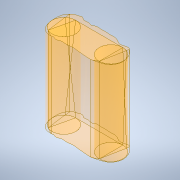
# Autodesk Inventor part: Kapton
Saved by Autodesk Inventor 2022 (Build 260153070, 153G)
## iProperties
Created: 2021-07-29
Part Number: Kapton
Material: Generic
Document SubType Name: Modeling
Designer: LJ
Density: 1 g/cm^3
Appearance: Default
Author: LJ
Autodesk Inventor part; units mm, degrees
ref_plane "Work Plane1" through (-0.6489, 57.7553, -49.1793) normal (0.0017309, 0.9999946, 0.0027762) x (0.9999985, -0.0017309, -0.0000024)
sketch "Sketch1" plane through (-0.6489, 57.7553, -49.1793) normal (0.0017309, 0.9999946, 0.0027762) x (0.9999985, -0.0017309, -0.0000024)
  circle A0 centre (0, 0) radius 9 projected
  line L0 (19.0189, 12.175) -> (12.9094, 12.175) projected
  line L1 (26.1347, 12.175) -> (20.0252, 12.175) projected
  circle A1 centre (36, 0) radius 9 projected
  circle A2 centre (18, 0) radius 9 projected
  spline S0 degree 4 poles (0, 0) (-0.6553, 0.9393) (-1.8109, 1.7925) (-2.0777, 3.7738) (-1.6084, 5.5868) (0.0105, 8.7964) (0.9505, 10.5382) (0.6689, 11.8602) (-0.5773, 12.0562) (-2.1364, 11.7342) (-4.3227, 10.9668) (-10.5073, 7.8875) (9.1877, 12.4202) (9.2116, 9.9398) knots 0 0 0 0 0 0.167802 0.242622 0.320476 0.395216 0.465981 0.526639 0.586559 0.652501 0.714955 1 1 1 1 1
  spline S1 degree 3 poles (35.4103, 0.0004) (35.5053, 0.524) (35.6027, 1.0612) (35.7334, 1.701) (35.99, 2.9576) (36.3593, 4.5369) (36.6244, 5.9708) (36.7554, 6.679) (36.8608, 7.3512) (36.9147, 7.9277) (36.9673, 8.4903) (36.9707, 8.9611) (36.9028, 9.2875) (36.8521, 9.5311) (36.762, 9.6946) (36.6361, 9.8005) (36.389, 10.0085) (36.0016, 9.9887) (35.5014, 9.8829) (34.889, 9.7534) (34.1057, 9.4918) (33.2228, 9.3567) (32.3613, 9.2249) (31.4183, 9.2115) (30.4339, 9.5143) (29.8991, 9.6789) (29.2864, 9.9624) (28.6807, 10.2059) (28.3816, 10.3262) (28.0815, 10.437) (27.7825, 10.5121) (27.4908, 10.5853) (27.1939, 10.6199) (26.945, 10.5735) (26.7256, 10.5326) (26.5741, 10.4399) (26.4467, 10.3351) (26.3224, 10.2328) (26.2215, 10.1171) (26.1249, 10.0075) knots 0 0 0 0 0.19652 0.19652 0.19652 0.582438 0.582438 0.582438 0.773039 0.773039 0.773039 0.959041 0.959041 0.959041 1.097848 1.097848 1.097848 1.370415 1.370415 1.370415 1.704123 1.704123 1.704123 2.029777 2.029777 2.029777 2.206716 2.206716 2.206716 2.294104 2.294104 2.294104 2.379384 2.379384 2.379384 2.454566 2.454566 2.454566 2.527933 2.527933 2.527933 2.527933 projected
  spline S2 degree 4 poles (18, 0) (19.219, -4.6198) (19.0867, -7.2448) (20.0738, -9.5935) (21.8548, -9.2534) (22.8608, -8.7189) (24.3983, -7.9162) (26.6917, -7.7224) (27.5292, -6.6832) (28.0308, -6.9813) (29.1474, -9.3707) (30.1409, -10.5959) (30.8392, -10.3204) (31.406, -9.5273) (32.8657, -2.3393) (33.0213, -3.9488) (34.3133, -0.7406) (36, 0) knots 0 0 0 0 0 0.198178 0.245011 0.293097 0.34823 0.403604 0.454446 0.508041 0.557208 0.603331 0.65184 0.7072 0.763584 0.826147 1 1 1 1 1
  spline S3 degree 4 poles (0, 0) (0.316, -1.3141) (-0.4427, -2.1492) (1.5587, -4.8996) (1.1525, -5.5021) (6.9051, -10.347) (5.2306, -9.9563) (5.4718, -9.4308) (4.7958, -8.7149) (4.8713, -8.5892) (6.0233, -7.3868) (6.4249, -6.4273) (7.496, -5.0511) (7.9624, -4.7173) (8.5564, -4.544) (9.1281, -4.9199) (9.5442, -5.4892) (10.5497, -8.0062) (11.3864, -8.8266) (11.913, -9.0938) (12.5739, -9.1265) (13.2529, -8.8682) (14.0483, -8.3031) (14.9715, -7.3561) (15.9318, -6.1181) (17.1481, -4.1239) (17.8173, -2.3655) (17.8952, -1.0974) (18, 0) knots 0 0 0 0 0 0.106192 0.157046 0.202296 0.242489 0.278377 0.299002 0.324044 0.354605 0.389092 0.425776 0.458865 0.486598 0.510804 0.543347 0.579427 0.615676 0.650761 0.678071 0.704423 0.734584 0.769524 0.808892 0.851075 0.893896 1 1 1 1 1
  line L2 (45, 0) -> (-9, 0) construction
  line L3 (36.017, -8.983) -> (-0.017, -8.983)
  line L4 (-0.017, 8.983) -> (36.017, 8.983)
  arc A3 (36.017, -8.983) -> (36.017, 8.983) centre (36.017, 0) ccw
  arc A4 (-0.017, 8.983) -> (-0.017, -8.983) centre (-0.017, 0) ccw
  spline S4 degree 4 poles (36.017, -8.983) (30.9958, -11.8975) (32.9255, -10.9101) (20.3119, -10.7814) (17.0217, -9.4088) (11.9966, -11.0587) (7.7415, -9.3427) (4.9899, -13.2783) (-0.7034, -7.4236) (4.6474, -13.4212) (-4.0003, -8.0516) knots 0 0 0 0 0 0.248405 0.34954 0.4777 0.586934 0.689222 0.769465 1 1 1 1 1
  line L5 (33.2745, -11.2682) -> (27.229, -10.9748) construction
  arc A5 (27.87, -10.8242) -> (32.6511, -11.0562) centre (31.021, 4.731) ccw construction
  spline S5 degree 4 poles (39.4127, 8.3165) (40.3947, 14.1433) (33.3903, 7.9791) (31.0784, 10.9351) (26.568, 13.0803) (22.0016, 12.3238) (19.3951, 13.1286) (15.2242, 12.4193) (10.9289, 13.6735) (10.0964, 10.5112) (5.6837, 13.436) (3.1602, 10.8421) (0.6242, 14.7157) (-1.5277, 12.7493) (-4.2485, 12.8468) (-8.0804, 10.3045) (-5.1576, 8.6318) (-5.9436, 6.7582) knots 0 0 0 0 0 0.164251 0.230539 0.292753 0.357884 0.423213 0.483129 0.544452 0.602591 0.659384 0.716439 0.769779 0.822475 0.871652 1 1 1 1 1
  point P0 (0.7487, -49.3395)
  point P1 (-1.1248, 1.4068)
  point P2 (-1.7551, 2.6503)
  point P3 (-1.8869, 3.9631)
  point P4 (-1.5342, 5.4984)
  point P5 (0.1303, 9.0153)
  point P6 (0.7446, 10.8943)
  point P7 (0.4337, 11.6763)
  point P8 (-0.4454, 11.9522)
  point P9 (-1.9244, 11.748)
  point P10 (-3.6466, 11.1412)
  point P11 (-5.2484, 10.192)
  point P12 (-4.8281, 9.9378)
  point P13 (19.4937, -7.2805)
  point P14 (20.2025, -8.8191)
  point P15 (20.9141, -9.2849)
  point P16 (21.7005, -9.2325)
  point P17 (22.6829, -8.8114)
  point P18 (24.5254, -8.0465)
  point P19 (26.8142, -7.3575)
  point P20 (27.5256, -6.9369)
  point P21 (27.9025, -7.0716)
  point P22 (29.3016, -9.4309)
  point P23 (30.2518, -10.3642)
  point P24 (30.6575, -10.3112)
  point P25 (31.1154, -9.766)
  point P26 (32.4478, -4.8226)
  point P27 (33.0116, -3.3798)
  point P28 (33.7624, -2.1885)
  point P29 (0.1165, -1.7118)
  point P30 (0.4378, -3.1699)
  point P31 (1.1027, -4.6194)
  point P32 (2.0695, -6.0716)
  point P33 (5.441, -9.7641)
  point P34 (5.6866, -9.9388)
  point P35 (5.2926, -9.3609)
  point P36 (4.9377, -8.8207)
  point P37 (4.9168, -8.6025)
  point P38 (5.6622, -7.7066)
  point P39 (6.6193, -6.2565)
  point P40 (7.6429, -4.9923)
  point P41 (8.0944, -4.7038)
  point P42 (8.5096, -4.6419)
  point P43 (8.9285, -4.8206)
  point P44 (9.398, -5.3741)
  point P45 (10.7591, -8.0516)
  point P46 (11.559, -8.8787)
  point P47 (12.0061, -9.0622)
  point P48 (12.5129, -9.0802)
  point P49 (13.1221, -8.8868)
  point P50 (13.8878, -8.382)
  point P51 (14.8388, -7.4545)
  point P52 (15.86, -6.1538)
  point P53 (16.7814, -4.6401)
  point P54 (17.4543, -3.102)
  point P55 (17.8169, -1.6352)
  point P56 (18, 0)
  point P57 (30.2518, -11.1215)
  point P58 (20.8791, -10.3343)
  point P59 (16.3717, -9.9691)
  point P60 (11.5107, -10.3427)
  point P61 (7.5994, -10.3924)
  point P62 (4.8814, -11.175)
  point P63 (2.404, -10.3272)
  point P64 (2.0502, -10.3236)
  point P65 (37.3714, 11.1319)
  point P66 (32.4445, 10.1835)
  point P67 (29.6646, 11.3962)
  point P68 (26.4295, 12.6021)
  point P69 (22.2745, 12.6345)
  point P70 (19.1979, 12.8254)
  point P71 (14.8368, 12.8262)
  point P72 (11.3002, 12.6682)
  point P73 (9.5875, 11.7437)
  point P74 (5.94, 12.3522)
  point P75 (3.0221, 12.1719)
  point P76 (0.4369, 13.622)
  point P77 (-1.5349, 13.1224)
  point P78 (-3.6471, 12.5265)
  point P79 (-5.9261, 11.1402)
  point P80 (-6.2045, 9.4639)
  point P81 (39.4145, 8.3271)
  point P82 (0.5527, 8.983)
  point P83 (17.4473, 8.983)
  point P84 (18.5527, 8.983)
  point P85 (35.4473, 8.983)
  point P86 (-3.9193, -8.1018)
  point P87 (35.9877, -9)
  constraints: 12 point on circle, 10 end point, 4 tangent, 3 centre point, 3 midpoint, 2 point on line, 1 horizontal, 1 parallel, 152 other
sketch "Sketch2" plane through (0, 0, 0) normal (1, 0, 0) x (0, 1, 0)
  point P0 (0, 0)
ref_plane "Work Plane2" through (35.2391, -7.0067, -49.359) normal (-0.0017309, -0.9999946, -0.0027762) x (-0.9999985, 0.0017309, 0.0000024)
sketch "Sketch3" plane through (35.2391, -7.0067, -49.359) normal (-0.0017309, -0.9999946, -0.0027762) x (-0.9999985, 0.0017309, 0.0000024)
  circle A0 centre (0, 0) radius 9
  line L0 (36.017, 8.983) -> (-0.017, 8.983) projected
  circle A1 centre (36, 0) radius 9
  line L1 (-0.017, -8.983) -> (36.017, -8.983) projected
  spline S0 degree 4 poles (-0.017, -8.983) (5.0042, -11.8975) (3.0745, -10.9101) (15.6881, -10.7814) (18.9783, -9.4088) (24.0034, -11.0587) (28.2585, -9.3427) (31.0101, -13.2783) (36.7034, -7.4236) (31.3526, -13.4212) (40.0003, -8.0516) knots 0 0 0 0 0 0.248405 0.34954 0.4777 0.586934 0.689222 0.769465 1 1 1 1 1 projected
  point P0 (35.2513, -49.3395)
  constraints: 2 centre point
sketch3d "3D Sketch1"
sketch "Sketch4" plane through (-0.6489, 57.7553, -49.1793) normal (0.0017309, 0.9999946, 0.0027762) x (0.9999985, -0.0017309, -0.0000024)
  spline S0 degree 4 poles (39.4127, 8.3165) (40.3947, 14.1433) (33.3903, 7.9791) (31.0784, 10.9351) (26.568, 13.0803) (22.0016, 12.3238) (19.3951, 13.1286) (15.2242, 12.4193) (10.9289, 13.6735) (10.0964, 10.5112) (5.6837, 13.436) (3.1602, 10.8421) (0.6242, 14.7157) (-1.5277, 12.7493) (-4.2485, 12.8468) (-8.0804, 10.3045) (-5.1576, 8.6318) (-5.9436, 6.7582) knots 0 0 0 0 0 0.164251 0.230539 0.292753 0.357884 0.423213 0.483129 0.544452 0.602591 0.659384 0.716439 0.769779 0.822475 0.871652 1 1 1 1 1 projected
  circle A0 centre (36, 0) radius 9 projected
  spline S1 degree 4 poles (36.017, -8.983) (30.9958, -11.8975) (32.9255, -10.9101) (20.3119, -10.7814) (17.0217, -9.4088) (11.9966, -11.0587) (7.7415, -9.3427) (4.9899, -13.2783) (-0.7034, -7.4236) (4.6474, -13.4212) (-4.0003, -8.0516) knots 0 0 0 0 0 0.248405 0.34954 0.4777 0.586934 0.689222 0.769465 1 1 1 1 1 projected
  circle A1 centre (0, 0) radius 9 projected
  point P0 (0.7487, -49.3395)
  constraints: 1 other
extrude "Extrusion2" add sketch "Sketch1" against normal up to surface (64.7 mm away)
surface_loft "LoftSrf1"
surface_loft "LoftSrf2"
surface_loft "LoftSrf3"
surface_loft "LoftSrf4"
boundary_patch "Boundary Patch1"
boundary_patch "Boundary Patch2"
boundary_patch "Boundary Patch3"
boundary_patch "Boundary Patch4"
boundary_patch "Boundary Patch5"
feature "Trim1" [suppressed]
feature "Trim2" [suppressed]
feature "Trim3" [suppressed]
ref_plane "Work Plane3" through (35.2951, 25.3431, -49.2692) normal (-0.0017309, -0.9999946, -0.0027762) x (0.9999985, -0.0017309, 0)
mirror "Mirror1" about plane through (35.2951, 25.3431, -49.2692) normal (-0.0017309, -0.9999946, -0.0027762) of "LoftSrf3", "LoftSrf1", "Boundary Patch3", "Boundary Patch1"
sketch "Sketch5" plane through (-0.6489, 57.7553, -49.1793) normal (-0.0017309, -0.9999946, -0.0027762) x (0.9999985, -0.0017309, 0)
  circle A0 centre (0, 0) radius 9 projected
  circle A1 centre (0, 0) radius 9 projected
  spline S0 degree 4 poles (-6.1806, -10.6808) (-11.3244, -6.7161) (-8.1732, 0.3491) (-10.5194, 11.463) (1.3876, 10.6993) knots 0 0 0 0 0 1 1 1 1 1
  point P0 (0.7489, 49.3395)
  point P1 (-8.7595, -6.4978)
  point P2 (-9, 0)
  point P3 (-6.8579, 7.1286)
  constraints: 1 point on circle, 10 other
sketch "Sketch6" plane through (-0.7609, -6.9444, -49.3589) normal (0.0017309, 0.9999946, 0.0027762) x (0.9999985, -0.0017309, 0)
  spline S0 degree 4 poles (-6.1806, 10.6808) (-11.3244, 6.7161) (-8.1732, -0.3491) (-10.5194, -11.463) (1.3876, -10.6993) knots 0 0 0 0 0 1 1 1 1 1 projected
  circle A0 centre (0, 0) radius 9 projected
  point P0 (0.7489, -49.3395)
  constraints: 3 other
surface_loft "LoftSrf7"
sketch "Sketch7" plane through (35.351, 57.693, -49.1794) normal (-0.0017309, -0.9999946, -0.0027762) x (0.9999985, -0.0017309, 0)
  circle A0 centre (0, 0) radius 9 projected
  spline S0 degree 4 poles (3.4145, -10.3622) (5.173, -9.6889) (13.8697, -0.6461) (7.1145, 8.7498) (3.058, 9.3295) (-4.3085, 11.0718) knots 0 0 0 0 0 0.478272 1 1 1 1 1
  point P0 (-35.2511, 49.3395)
  point P1 (6.9331, -7.0444)
  point P2 (9.3606, -0.0002)
  point P3 (7.8001, 5.3532)
  point P4 (4.679, 8.3442)
  constraints: 11 other
sketch "Sketch8" plane through (35.2391, -7.0067, -49.359) normal (0.0017309, 0.9999946, 0.0027762) x (0.9999985, -0.0017309, 0)
  spline S0 degree 4 poles (3.4145, 10.3622) (5.173, 9.6889) (13.8697, 0.6461) (7.1145, -8.7498) (3.058, -9.3295) (-4.3085, -11.0718) knots 0 0 0 0 0 0.478272 1 1 1 1 1 projected
  circle A0 centre (0, 0) radius 9 projected
  point P0 (-35.2511, -49.3395)
  constraints: 3 other
surface_loft "LoftSrf8"
body "Solid2"
body "Srf1"
body "Srf2"
body "Srf3"
body "Srf4"
body "Srf5"
body "Srf6"
body "Srf7"
body "Srf8"
body "Srf9"
body "Srf10"
body "Srf11"
body "Srf12"
body "Srf13"
body "Srf14"
body "Srf15"
